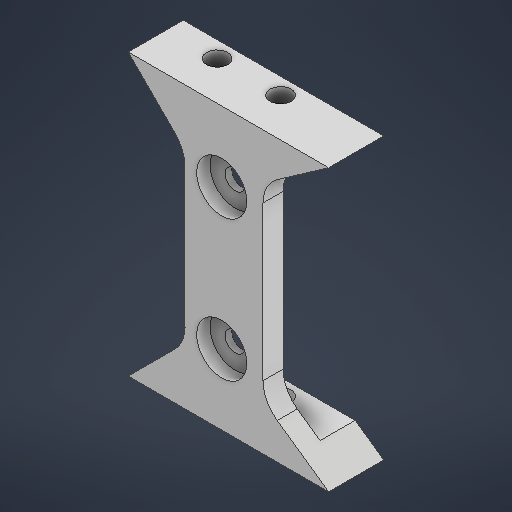
# Autodesk Inventor part: horni_kloub_extenze_drzak
Saved by Autodesk Inventor 2026 (Build 300175000, 175)
## iProperties
Created: 2025-04-11
Part Number: horni_kloub_extenze_drzak
Material: Generic
Document SubType Name: Modeling
Designer: janpa
Density: 1 g/cm^3
Appearance: Default
Author: janpa
Autodesk Inventor part; units mm, degrees
ref_plane "YZ Plane" through (0, 0, 0) normal (1, 0, 0) x (0, 1, 0)
ref_plane "XZ Plane" through (0, 0, 0) normal (0, 1, 0) x (-1, 0, 0)
ref_plane "XY Plane" through (0, 0, 0) normal (0, 0, 1) x (1, 0, 0)
sketch "Sketch1" plane through (0, 0, 0) normal (1, 0, 0) x (0, 1, 0)
  line L0 (0, 0) -> (42, 0)
  line L1 (42, 0) -> (42, 3)
  line L2 (42, 3) -> (0, 3)
  line L3 (0, 3) -> (0, 0)
  line L4 (42, 3) -> (39, 3)
  line L5 (39, 3) -> (39, -5.25)
  line L6 (39, -5.25) -> (42, -5.25)
  line L7 (42, -5.25) -> (42, 3)
  line L8 (21, 3) -> (21, 5.7784)
  line L9 (42, 0) -> (0, 0)
  line L10 (0, 0) -> (0, 3)
  line L11 (0, 3) -> (42, 3)
  line L12 (0, 3) -> (3, 3)
  line L13 (3, 3) -> (3, -5.25)
  line L14 (3, -5.25) -> (0, -5.25)
  line L15 (0, -5.25) -> (0, 3)
  point P0 (3, 0)
  point P1 (39, 0)
  dimension "d0" = 42
  dimension "d1" = 3
  dimension "d2" = 3
  dimension "d3" = 8.25
  constraints: 32 end point, 7 symmetric about line, 4 parallel, 2 horizontal, 2 perpendicular, 1 midpoint, 1 vertical
  measures "d0" distance of L2.end L1.end
  measures "d1" distance of L1.end L0.end
  measures "d2" distance of L6.end L5.end
  measures "d3" distance of L5.end L4.end
extrude "Extrusion1" add sketch "Sketch1" along normal blind 30
sketch "Sketch2" plane through (0, 0, -5.25) normal (0, -1, 0) x (1, 0, 0)
  circle A0 centre (17, 2.45) radius 1.5875
  line L0 (30, 8.25) -> (30, 0) projected
  line L1 (0, 8.25) -> (30, 8.25) projected
  line L2 (0, 0) -> (30, 0) projected
  circle A1 centre (7.5, 2.45) radius 1.5875
  point P0 (0, 5.25)
  dimension "d7" = 5.8
  dimension "d8" = 9.5
  dimension "d35" = 13
  constraints: 2 centre point
  measures "d7" distance from line of L1 A0.centre
  measures "d8" distance of A0.centre A1.centre
  measures "d35" distance from line of L0 A0.centre
extrude "Extrusion2" cut sketch "Sketch2" against normal blind 60
sketch "Sketch3" plane through (0, 0, 3) normal (0, 0, 1) x (1, 0, 0)
  circle A0 centre (14, 31.5) radius 3.75
  circle A1 centre (14, 10.5) radius 3.75
  line L0 (30, 42) -> (30, 0) projected
  line L1 (0, 42) -> (0, 0) projected
  line L2 (0, 42) -> (30, 42) projected
  line L3 (0, 0) -> (30, 0) projected
  circle A2 centre (14, 31.5) radius 1.5
  circle A3 centre (14, 10.5) radius 1.5
  dimension "d11" = 7.5
  dimension "d12" = 7.5
  dimension "d13" = 16
  dimension "d14" = 14
  dimension "d15" = 16
  dimension "d16" = 10.5
  dimension "d17" = 10.5
  dimension "d20" = 3
  dimension "d21" = 3
  constraints: 4 centre point, 2 coincident
  measures "d11" diameter of A1
  measures "d12" diameter of A0
  measures "d13" distance from line of L0 A1.centre
  measures "d14" distance from line of L1 A1.centre
  measures "d15" distance from line of L0 A0.centre
  measures "d16" distance from line of L2 A0.centre
  measures "d17" distance from line of L3 A1.centre
  measures "d20" diameter of A2
  measures "d21" diameter of A3
extrude "Extrusion3" cut sketch "Sketch3" against normal blind 2 contours A0 | A1 | A2 | A3
extrude "Extrusion4" cut sketch "Sketch3" against normal blind 10 contours A2 | A3
sketch "Sketch4" plane through (0, 0, 3) normal (0, 0, 1) x (1, 0, 0)
  line L0 (0, 0) -> (7.0208, 7.0208)
  line L1 (0, 0) -> (9.9289, 0) construction
  line L2 (8.4853, 10.5563) -> (8.4853, 31.4437)
  line L3 (0, 42) -> (0, 0) projected
  line L4 (0, 42) -> (7.0208, 34.9792)
  line L5 (0, 42) -> (9.9289, 42) construction
  line L6 (0, 0) -> (30, 0) projected
  line L7 (30, 0) -> (22.3023, 5.39)
  line L8 (30, 0) -> (39.3972, 0) construction
  line L9 (30, 42) -> (22.3023, 36.61)
  line L10 (30, 42) -> (39.3972, 42) construction
  line L11 (20.1702, 32.5142) -> (20.1702, 9.4858)
  line L12 (8.4853, 33.5147) -> (8.4853, 32.6445)
  arc A0 (20.1702, 9.4858) -> (22.3023, 5.39) centre (25.1702, 9.4858) ccw
  arc A1 (22.3023, 36.61) -> (20.1702, 32.5142) centre (25.1702, 32.5142) ccw
  arc A2 (8.4853, 31.4437) -> (7.0208, 34.9792) centre (3.4853, 31.4437) ccw
  arc A3 (7.0208, 7.0208) -> (8.4853, 10.5563) centre (3.4853, 10.5563) ccw
  line L13 (30, 42) -> (30, 0) projected
  line L14 (30, 0) -> (30, 42)
  point P0 (8.4853, 8.4853)
  point P1 (20.1702, 6.8829)
  point P2 (20.1702, 35.1171)
  dimension "d24" = 12
  dimension "d25" = 45
  dimension "d26" = 12
  dimension "d27" = 45
  dimension "d28" = 12
  dimension "d29" = 145
  dimension "d30" = 12
  dimension "d31" = 145
  dimension "d32" = 5
  constraints: 24 end point, 8 point on circle, 8 point on line, 8 tangent, 4 centre point, 4 equal length, 4 horizontal, 3 equal radius, 1 collinear, 1 vertical
  measures "d24" distance of L0.start point (8.485, 8.485)
  measures "d25" angle of L1 L0
  measures "d26" distance of L3.start L12.start
  measures "d27" angle of L4 L5
  measures "d28" distance of L6.end point (20.17, 6.883)
  measures "d29" angle of L8 L7
  measures "d30" distance of L9.start point (20.17, 35.117)
  measures "d31" angle of L9 L10
  measures "d32" radius of A0
extrude "Extrusion5" cut sketch "Sketch4" against normal blind 10
body "Solid1"
